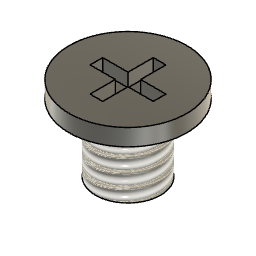
PSD Sun Sensor (Autodesk Fusion 360 archive; units mm, degrees)
design "M2x2 D3.5x0.5"
Autodesk Fusion 360 part; units mm, degrees
sketch "Sketch1" plane through (0, 0, 0) normal (0, 0, 1) x (1, 0, 0)
  circle A0 centre (0, 0) radius 1
  dimension "d1" = 2
  constraint coincident A0.centre origin
  measures "d1" diameter of A0
extrude "Extrude1" add sketch "Sketch1" against normal blind 2
sketch "Sketch2" plane through (0, 0, 0) normal (0, 0, 1) x (1, 0, 0)
  circle A0 centre (0, 0) radius 1.75
  dimension "d4" = 3.5
  constraint coincident A0.centre origin
  measures "d4" diameter of A0
extrude "Extrude2" add sketch "Sketch2" along normal blind 0.5
thread "Thread1" "ISO Metric profile 2.0 M2x0.4 6g" major diameter 1.9335 minor diameter 1.478 pitch 0.4 angle 60 resizes the face on face at (0.9988, -0.0498, -1.3333)
sketch "Sketch3" plane through (0, 0, 0.5) normal (0, 0, 1) x (-1, 0, 0)
  circle A0 centre (0, 0) radius 1.75
  line L0 (-0.9401, -0.188) -> (0.9401, -0.188)
  line L1 (0.9401, -0.188) -> (0.9401, 0.188)
  line L2 (0.9401, 0.188) -> (-0.9401, 0.188)
  line L3 (-0.9401, 0.188) -> (-0.9401, -0.188)
  line L4 (-0.9401, -0.188) -> (0.9401, 0.188) construction
  line L5 (0.9401, -0.188) -> (-0.9401, 0.188) construction
  line L6 (-0.188, -0.9401) -> (0.188, -0.9401)
  line L7 (0.188, -0.9401) -> (0.188, 0.9401)
  line L8 (0.188, 0.9401) -> (-0.188, 0.9401)
  line L9 (-0.188, 0.9401) -> (-0.188, -0.9401)
  line L10 (-0.188, -0.9401) -> (0.188, 0.9401) construction
  line L11 (0.188, -0.9401) -> (-0.188, 0.9401) construction
  constraint horizontal L0
  constraint perpendicular L0 L1
  constraint parallel L0 L2
  constraint parallel L1 L3
  constraint coincident L4 A0.centre
  constraint coincident L5 A0.centre
  constraint coincident A0.centre origin
  constraint horizontal L6
  constraint perpendicular L6 L7
  constraint parallel L6 L8
  constraint parallel L7 L9
  constraint coincident L10 A0.centre
  constraint coincident L11 A0.centre
  constraint equal L3 L6
  constraint equal L0 L9
extrude "Extrude3" cut sketch "Sketch3" against normal blind 0.4 contours L0 L2 L3 L9 | L0 L2 L7 L9 | L0 L6 L7 L9 | L0 L1 L2 L7 | L2 L7 L8 L9

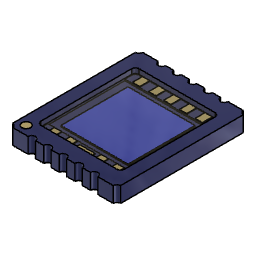
design "Hamamatsu S5990-01"
Autodesk Fusion 360 part; units mm, degrees
sketch "Sketch1" plane through (0, 0, 0) normal (0, 0, 1) x (1, 0, 0)
  line L0 (4.4, 5.3) -> (-4.4, 5.3)
  line L1 (-4.4, 5.3) -> (-4.4, -5.3)
  line L2 (-4.4, -5.3) -> (4.4, -5.3)
  line L3 (4.4, -5.3) -> (4.4, 5.3)
  line L4 (4.4, 5.3) -> (-4.4, -5.3) construction
  line L5 (-4.4, 5.3) -> (4.4, -5.3) construction
  circle A0 centre (-4.4, 5.3) radius 0.3
  circle A1 centre (4.4, 5.3) radius 0.3
  circle A2 centre (-4.4, -5.3) radius 0.3
  circle A3 centre (4.4, -5.3) radius 0.3
  dimension "d1" = 8.8
  dimension "d2" = 10.6
  dimension "d3" = 0.6
  constraint horizontal L0
  constraint perpendicular L0 L1
  constraint parallel L0 L2
  constraint parallel L1 L3
  constraint coincident L4 origin
  constraint coincident L5 origin
  constraint coincident L0.end L1.start
  constraint coincident L0.start L3.end
  constraint coincident L1.end L2.start
  constraint coincident L2.end L3.start
  constraint equal A1 A3
  constraint equal A2 A3
  constraint equal A0 A2
  measures "d1" distance of L1.end L2.end
  measures "d2" distance of L0.end L1.end
  measures "d3" diameter of A0
extrude "Extrude1" add sketch "Sketch1" along normal blind 1.26 contours L0 L1 L2 L3 A0 A1 A2 A3 makes body 1
sketch "Sketch2" plane through (0, 0, 1.26) normal (0, 0, 1) x (-1, 0, 0)
  line L0 (4.4, -5) -> (4.4, 5)
  arc A0 (4.1, 5.3) -> (4.4, 5) centre (4.4, 5.3) ccw
  line L1 (4.1, 5.3) -> (-4.1, 5.3)
  arc A1 (-4.4, 5) -> (-4.1, 5.3) centre (-4.4, 5.3) ccw
  line L2 (-4.4, 5) -> (-4.4, -5)
  arc A2 (-4.1, -5.3) -> (-4.4, -5) centre (-4.4, -5.3) ccw
  line L3 (-4.1, -5.3) -> (4.1, -5.3)
  arc A3 (4.4, -5) -> (4.1, -5.3) centre (4.4, -5.3) ccw
  line L4 (-3.4, -4) -> (3.4, -4)
  line L5 (3.4, -4) -> (3.4, 4)
  line L6 (3.4, 4) -> (-3.4, 4)
  line L7 (-3.4, 4) -> (-3.4, -4)
  line L8 (-3.4, -4) -> (3.4, 4) construction
  line L9 (3.4, -4) -> (-3.4, 4) construction
  dimension "d6" = 1
  dimension "d7" = 1.3
  constraint horizontal L4
  constraint perpendicular L4 L5
  constraint parallel L4 L6
  constraint parallel L5 L7
  constraint coincident L8 origin
  constraint coincident L9 origin
  measures "d6" distance of L0 L5
  measures "d7" distance of L3 L4
extrude "Extrude2" cut sketch "Sketch2" against normal blind 0.46 contours L4 L5 L6 L7 bodies 1
sketch "Sketch3" plane through (0, 0, 0.8) normal (0, 0, 1) x (-1, 0, 0)
  line L0 (-3.4, 4) -> (-3.4, -4)
  line L1 (-3.4, -4) -> (3.4, -4)
  line L2 (3.4, -4) -> (3.4, 4)
  line L3 (3.4, 4) -> (-3.4, 4)
  line L4 (-3.4, -3.1358) -> (3.4, -3.1358)
  line L5 (3.4, -3.1358) -> (3.4, 3.1358)
  line L6 (3.4, 3.1358) -> (-3.4, 3.1358)
  line L7 (-3.4, 3.1358) -> (-3.4, -3.1358)
  line L8 (-3.4, -3.1358) -> (3.4, 3.1358) construction
  line L9 (3.4, -3.1358) -> (-3.4, 3.1358) construction
  constraint horizontal L4
  constraint perpendicular L4 L5
  constraint parallel L4 L6
  constraint parallel L5 L7
  constraint coincident L8 origin
  constraint coincident L9 origin
  constraint coincident L0 L4.start
sketch "Sketch6" plane through (0, 0, 0.8) normal (0, 0, 1) x (-1, 0, 0)
  line L0 (-3.4, 4) -> (-3.4, -4)
  line L1 (-3.4, -4) -> (3.4, -4)
  line L2 (3.4, -4) -> (3.4, 4)
  line L3 (3.4, 4) -> (-3.4, 4)
  line L4 (2.8165, -4) -> (2.2221, -4)
  line L5 (2.2221, -4) -> (2.2221, -3.1841)
  line L6 (2.2221, -3.1841) -> (2.8165, -3.1841)
  line L7 (2.8165, -3.1841) -> (2.8165, -4)
  line L8 (1.5027, -4) -> (0.9082, -4)
  line L9 (0.9082, -4) -> (0.9082, -3.1841)
  line L10 (0.9082, -3.1841) -> (1.5027, -3.1841)
  line L11 (1.5027, -3.1841) -> (1.5027, -4)
  line L12 (0.2802, -4) -> (-0.3143, -4)
  line L13 (-0.3143, -4) -> (-0.3143, -3.1841)
  line L14 (-0.3143, -3.1841) -> (0.2802, -3.1841)
  line L15 (0.2802, -3.1841) -> (0.2802, -4)
  line L16 (-1.007, -4) -> (-1.6015, -4)
  line L17 (-1.6015, -4) -> (-1.6015, -3.1841)
  line L18 (-1.6015, -3.1841) -> (-1.007, -3.1841)
  line L19 (-1.007, -3.1841) -> (-1.007, -4)
  line L20 (-2.2803, -4) -> (-2.8747, -4)
  line L21 (-2.8747, -4) -> (-2.8747, -3.1841)
  line L22 (-2.8747, -3.1841) -> (-2.2803, -3.1841)
  line L23 (-2.2803, -3.1841) -> (-2.2803, -4)
  line L24 (2.8085, 4) -> (2.2141, 4)
  line L25 (2.2141, 4) -> (2.2141, 3.1841)
  line L26 (2.2141, 3.1841) -> (2.8085, 3.1841)
  line L27 (2.8085, 3.1841) -> (2.8085, 4)
  line L28 (1.5132, 4) -> (0.9187, 4)
  line L29 (0.9187, 4) -> (0.9187, 3.1841)
  line L30 (0.9187, 3.1841) -> (1.5132, 3.1841)
  line L31 (1.5132, 3.1841) -> (1.5132, 4)
  line L32 (-1.0056, 4) -> (-1.6, 4)
  line L33 (-1.6, 4) -> (-1.6, 3.1841)
  line L34 (-1.6, 3.1841) -> (-1.0056, 3.1841)
  line L35 (-1.0056, 3.1841) -> (-1.0056, 4)
  line L36 (0.5753, 4) -> (-0.7, 4)
  line L37 (-0.7, 4) -> (-0.7, 3.3622)
  line L38 (-0.7, 3.3622) -> (0.5753, 3.3622)
  line L39 (0.5753, 3.3622) -> (0.5753, 4)
  line L40 (-2.2961, 4) -> (-2.8905, 4)
  line L41 (-2.8905, 4) -> (-2.8905, 3.1841)
  line L42 (-2.8905, 3.1841) -> (-2.2961, 3.1841)
  line L43 (-2.2961, 3.1841) -> (-2.2961, 4)
  constraint horizontal L4
  constraint vertical L5
  constraint horizontal L6
  constraint vertical L7
  constraint coincident L1 L4.start
  constraint horizontal L8
  constraint vertical L9
  constraint horizontal L10
  constraint vertical L11
  constraint coincident L1 L8.start
  constraint horizontal L12
  constraint vertical L13
  constraint horizontal L14
  constraint vertical L15
  constraint coincident L1 L12.start
  constraint horizontal L16
  constraint vertical L17
  constraint horizontal L18
  constraint vertical L19
  constraint coincident L1 L16.start
  constraint horizontal L20
  constraint vertical L21
  constraint horizontal L22
  constraint vertical L23
  constraint coincident L1 L20.start
  constraint equal L19 L23
  constraint equal L15 L19
  constraint equal L11 L15
  constraint equal L7 L11
  constraint equal L6 L10
  constraint equal L10 L14
  constraint equal L14 L18
  constraint equal L18 L22
  constraint horizontal L24
  constraint vertical L25
  constraint horizontal L26
  constraint vertical L27
  constraint coincident L3 L24.start
  constraint horizontal L28
  constraint vertical L29
  constraint horizontal L30
  constraint vertical L31
  constraint coincident L3 L28.start
  constraint horizontal L32
  constraint vertical L33
  constraint horizontal L34
  constraint vertical L35
  constraint coincident L3 L32.start
  constraint horizontal L36
  constraint vertical L37
  constraint horizontal L38
  constraint vertical L39
  constraint coincident L3 L36.start
  constraint horizontal L40
  constraint vertical L41
  constraint horizontal L42
  constraint vertical L43
  constraint coincident L3 L40.start
  constraint equal L34 L42
  constraint equal L30 L42
  constraint equal L26 L30
  constraint equal L6 L26
  constraint equal L27 L31
  constraint equal L7 L31
  constraint equal L7 L35
  constraint equal L35 L43
extrude "Extrude1'" add sketch "Sketch6" along normal blind 0.05 separate body contours L3 L40 L41 L42 L43 | L1 L20 L21 L22 L23 | L3 L32 L33 L34 L35 | L1 L16 L17 L18 L19 | L3 L36 L37 L38 L39 | L1 L12 L13 L14 L15 | L3 L28 L29 L30 L31 | L1 L8 L9 L10 L11 | L3 L24 L25 L26 L27 | L1 L4 L5 L6 L7 makes body 2 at (-0.082, 3.728, 0.8) makes body 3 at (1.4019, -3.728, 0.8) makes body 4 at (-2.4123, -3.728, 0.8) makes body 5 at (2.4942, -3.728, 0.8) makes body 6 at (-1.1064, 3.4561, 0.8) makes body 7 at (1.4033, 3.4561, 0.8) makes body 8 at (0.2749, -3.7874, 0.8) makes body 9 at (-1.315, -3.4561, 0.8) makes body 10 at (2.6765, 3.4561, 0.8) makes body 11 at (-2.4202, 3.4561, 0.8) in component "Component"
extrude "Extrude3" cut sketch "Sketch3" against normal blind 0.1 contours L0 L2 L4 L5 L6 L7 bodies 1
sketch "Sketch4" plane through (0, 0, 0.7) normal (0, 0, 1) x (-1, 0, 0)
  line L0 (-3.4, 3.1358) -> (-3.4, -3.1358)
  line L1 (-3.4, -3.1358) -> (3.4, -3.1358)
  line L2 (3.4, -3.1358) -> (3.4, 3.1358)
  line L3 (3.4, 3.1358) -> (-3.4, 3.1358)
  line L4 (-2.734, -2.734) -> (2.734, -2.734)
  line L5 (2.734, -2.734) -> (2.734, 2.734)
  line L6 (2.734, 2.734) -> (-2.734, 2.734)
  line L7 (-2.734, 2.734) -> (-2.734, -2.734)
  line L8 (-2.734, -2.734) -> (2.734, 2.734) construction
  line L9 (2.734, -2.734) -> (-2.734, 2.734) construction
  constraint horizontal L4
  constraint perpendicular L4 L5
  constraint parallel L4 L6
  constraint parallel L5 L7
  constraint coincident L8 origin
  constraint coincident L9 origin
  constraint equal L4 L5
extrude "Extrude1''" add sketch "Sketch4" along normal blind 0.1 separate body contours L4 L5 L6 L7 makes body 12 in component "Diode"
fillet "Fillet1" radius 0.3 4 edges at (-3.4, 4, 1.03) (-3.4, -4, 1.03) (3.4, -4, 1.03) (3.4, 4, 1.03) on bodies 1
sketch "Sketch5" plane through (0, 0, 0) normal (0, 0, 1) x (1, 0, 0)
  line L0 (4.4, 5.3) -> (-4.4, 5.3)
  line L1 (-4.4, 5.3) -> (-4.4, -5.3)
  line L2 (-4.4, -5.3) -> (4.4, -5.3)
  line L3 (4.4, -5.3) -> (4.4, 5.3)
  circle A0 centre (0, 5.3) radius 0.3
  circle A1 centre (1.27, 5.3) radius 0.3
  circle A2 centre (2.54, 5.3) radius 0.3
  circle A3 centre (-1.27, 5.3) radius 0.3
  circle A4 centre (-2.54, 5.3) radius 0.3
  circle A5 centre (0, -5.3) radius 0.3
  circle A6 centre (1.27, -5.3) radius 0.3
  circle A7 centre (2.54, -5.3) radius 0.3
  circle A8 centre (-1.27, -5.3) radius 0.3
  circle A9 centre (-2.54, -5.3) radius 0.3
  line L4 (-2.84, 5.3) -> (-2.24, 5.3)
  line L5 (-2.24, 5.3) -> (-2.24, 3.8)
  line L6 (-2.24, 3.8) -> (-2.84, 3.8)
  line L7 (-2.84, 3.8) -> (-2.84, 5.3)
  line L8 (-1.57, 5.3) -> (-0.97, 5.3)
  line L9 (-0.97, 5.3) -> (-0.97, 3.8)
  line L10 (-0.97, 3.8) -> (-1.57, 3.8)
  line L11 (-1.57, 3.8) -> (-1.57, 5.3)
  line L12 (-0.3, 5.3) -> (0.3, 5.3)
  line L13 (0.3, 5.3) -> (0.3, 3.8)
  line L14 (0.3, 3.8) -> (-0.3, 3.8)
  line L15 (-0.3, 3.8) -> (-0.3, 5.3)
  line L16 (0.97, 5.3) -> (1.57, 5.3)
  line L17 (1.57, 5.3) -> (1.57, 3.8)
  line L18 (1.57, 3.8) -> (0.97, 3.8)
  line L19 (0.97, 3.8) -> (0.97, 5.3)
  line L20 (2.24, 5.3) -> (2.84, 5.3)
  line L21 (2.84, 5.3) -> (2.84, 3.8)
  line L22 (2.84, 3.8) -> (2.24, 3.8)
  line L23 (2.24, 3.8) -> (2.24, 5.3)
  line L24 (-2.84, -5.3) -> (-2.24, -5.3)
  line L25 (-2.24, -5.3) -> (-2.24, -3.8)
  line L26 (-2.24, -3.8) -> (-2.84, -3.8)
  line L27 (-2.84, -3.8) -> (-2.84, -5.3)
  line L28 (-1.57, -5.3) -> (-0.97, -5.3)
  line L29 (-0.97, -5.3) -> (-0.97, -3.8)
  line L30 (-0.97, -3.8) -> (-1.57, -3.8)
  line L31 (-1.57, -3.8) -> (-1.57, -5.3)
  line L32 (-0.3, -5.3) -> (0.3, -5.3)
  line L33 (0.3, -5.3) -> (0.3, -2.8)
  line L34 (0.3, -2.8) -> (-0.3, -2.8)
  line L35 (-0.3, -2.8) -> (-0.3, -5.3)
  line L36 (0.97, -5.3) -> (1.57, -5.3)
  line L37 (1.57, -5.3) -> (1.57, -3.8)
  line L38 (1.57, -3.8) -> (0.97, -3.8)
  line L39 (0.97, -3.8) -> (0.97, -5.3)
  line L40 (2.24, -5.3) -> (2.84, -5.3)
  line L41 (2.84, -5.3) -> (2.84, -3.8)
  line L42 (2.84, -3.8) -> (2.24, -3.8)
  line L43 (2.24, -3.8) -> (2.24, -5.3)
  dimension "d17" = 0.6
  dimension "d18" = 1.27
  dimension "d19" = 1.27
  dimension "d20" = 1.27
  dimension "d21" = 1.27
  dimension "d22" = 1.27
  dimension "d23" = 1.27
  dimension "d24" = 1.27
  dimension "d25" = 1.27
  dimension "d26" = 1.5
  dimension "d38" = 2.5
  constraint midpoint L0 A0.centre
  constraint coincident L0 A1.centre
  constraint coincident L0 A2.centre
  constraint coincident L0 A3.centre
  constraint coincident L0 A4.centre
  constraint midpoint L2 A5.centre
  constraint coincident L2 A6.centre
  constraint coincident L2 A7.centre
  constraint coincident L2 A8.centre
  constraint coincident L2 A9.centre
  constraint equal A8 A9
  constraint equal A5 A9
  constraint equal A5 A6
  constraint equal A6 A7
  constraint equal A2 A7
  constraint equal A1 A2
  constraint equal A1 A3
  constraint equal A3 A4
  constraint equal A0 A4
  constraint perpendicular L4 L5
  constraint parallel L4 L6
  constraint parallel L5 L7
  constraint coincident A4 L4.end
  constraint coincident L0 L4.end
  constraint parallel L0 L4
  constraint coincident A4 L4.start
  constraint perpendicular L8 L9
  constraint parallel L8 L10
  constraint parallel L9 L11
  constraint coincident A3 L8.end
  constraint coincident L0 L8.end
  constraint perpendicular L7 L8
  constraint coincident A3 L8.start
  constraint perpendicular L12 L13
  constraint parallel L12 L14
  constraint parallel L13 L15
  constraint coincident A0 L12.end
  constraint coincident L0 L12.end
  constraint perpendicular L9 L12
  constraint coincident A0 L12.start
  constraint perpendicular L16 L17
  constraint parallel L16 L18
  constraint parallel L17 L19
  constraint coincident L0 L16.end
  constraint coincident A1 L16.end
  constraint perpendicular L13 L16
  constraint coincident A1 L16.start
  constraint perpendicular L20 L21
  constraint parallel L20 L22
  constraint parallel L21 L23
  constraint coincident A2 L20.end
  constraint coincident L0 L20.end
  constraint perpendicular L17 L20
  constraint coincident A2 L20.start
  constraint perpendicular L24 L25
  constraint parallel L24 L26
  constraint parallel L25 L27
  constraint coincident A9 L24.end
  constraint coincident L2 L24.end
  constraint perpendicular L23 L24
  constraint coincident A9 L24.start
  constraint perpendicular L28 L29
  constraint parallel L28 L30
  constraint parallel L29 L31
  constraint coincident A8 L28.end
  constraint coincident L2 L28.end
  constraint perpendicular L27 L28
  constraint coincident A8 L28.start
  constraint perpendicular L32 L33
  constraint parallel L32 L34
  constraint parallel L33 L35
  constraint coincident A5 L32.end
  constraint coincident L2 L32.end
  constraint perpendicular L29 L32
  constraint coincident A5 L32.start
  constraint perpendicular L36 L37
  constraint parallel L36 L38
  constraint parallel L37 L39
  constraint coincident A6 L36.end
  constraint coincident L2 L36.end
  constraint perpendicular L33 L36
  constraint coincident A6 L36.start
  constraint perpendicular L40 L41
  constraint parallel L40 L42
  constraint parallel L41 L43
  constraint coincident A7 L40.end
  constraint coincident L2 L40.end
  constraint perpendicular L39 L40
  constraint coincident A7 L40.start
  constraint equal L7 L11
  constraint equal L11 L19
  constraint equal L19 L23
  constraint equal L23 L27
  constraint equal L27 L31
  constraint equal L39 L43
  constraint equal L11 L15
  constraint equal L31 L39
  measures "d17" diameter of A0
  measures "d18" distance of A0.centre A3.centre
  measures "d19" distance of A0.centre A1.centre
  measures "d20" distance of A1.centre A2.centre
  measures "d21" distance of A3.centre A4.centre
  measures "d22" distance of A5.centre A8.centre
  measures "d23" distance of A8.centre A9.centre
  measures "d24" distance of A5.centre A6.centre
  measures "d25" distance of A6.centre A7.centre
  measures "d26" distance of A4.centre L6
  measures "d38" distance of A5.centre L34
extrude "Extrude5" cut sketch "Sketch5" along normal blind 1.5 contours L0 A2 L20 | L2 A7 L40 | L0 A1 L16 | L2 A6 L36 | L0 A0 L12 | L2 A5 L32 | L0 A3 L8 | L2 A8 L28 | L0 A4 L4 | L2 A9 L24 picked at (2.5697, 5.1028) picked at (2.6301, -5.2566) picked at (1.2077, 5.2218) picked at (1.3433, -5.232) picked at (-0.0623, 5.2218) picked at (-0.0989, -5.2851) picked at (-1.3323, 5.2218) picked at (-1.1967, -5.232) picked at (-2.5103, 5.1028) picked at (-2.4499, -5.2566) bodies 1
extrude "Extrude1'''" add sketch "Sketch2" against normal blind 0.4 separate body contours L4 L5 L6 L7 makes body 13 in component "Resin Window"
fillet "Fillet1'" radius 0.3 4 edges at (-3.4, -4, 1.06) (3.4, -4, 1.06) (3.4, 4, 1.06) (-3.4, 4, 1.06) on bodies 13 in component "Resin Window"
sketch "Sketch7" plane through (0, 0, 1.26) normal (0, 0, 1) x (-1, 0, 0)
  arc A0 (0.3, -5.3) -> (-0.3, -5.3) centre (0, -5.3) ccw
  line L0 (0.3, -5.3) -> (0.97, -5.3)
  arc A1 (1.57, -5.3) -> (0.97, -5.3) centre (1.27, -5.3) ccw
  line L1 (1.57, -5.3) -> (2.24, -5.3)
  arc A2 (2.84, -5.3) -> (2.24, -5.3) centre (2.54, -5.3) ccw
  line L2 (2.84, -5.3) -> (4.1, -5.3)
  arc A3 (4.4, -5) -> (4.1, -5.3) centre (4.4, -5.3) ccw
  line L3 (4.4, -5) -> (4.4, 5)
  arc A4 (4.1, 5.3) -> (4.4, 5) centre (4.4, 5.3) ccw
  line L4 (4.1, 5.3) -> (2.84, 5.3)
  arc A5 (2.24, 5.3) -> (2.84, 5.3) centre (2.54, 5.3) ccw
  line L5 (2.24, 5.3) -> (1.57, 5.3)
  arc A6 (0.97, 5.3) -> (1.57, 5.3) centre (1.27, 5.3) ccw
  line L6 (0.97, 5.3) -> (0.3, 5.3)
  arc A7 (-0.3, 5.3) -> (0.3, 5.3) centre (0, 5.3) ccw
  line L7 (-0.3, 5.3) -> (-0.97, 5.3)
  arc A8 (-1.57, 5.3) -> (-0.97, 5.3) centre (-1.27, 5.3) ccw
  line L8 (-1.57, 5.3) -> (-2.24, 5.3)
  arc A9 (-2.84, 5.3) -> (-2.24, 5.3) centre (-2.54, 5.3) ccw
  line L9 (-2.84, 5.3) -> (-4.1, 5.3)
  arc A10 (-4.4, 5) -> (-4.1, 5.3) centre (-4.4, 5.3) ccw
  line L10 (-4.4, 5) -> (-4.4, -5)
  arc A11 (-4.1, -5.3) -> (-4.4, -5) centre (-4.4, -5.3) ccw
  line L11 (-4.1, -5.3) -> (-2.84, -5.3)
  arc A12 (-2.24, -5.3) -> (-2.84, -5.3) centre (-2.54, -5.3) ccw
  line L12 (-2.24, -5.3) -> (-1.57, -5.3)
  arc A13 (-0.97, -5.3) -> (-1.57, -5.3) centre (-1.27, -5.3) ccw
  line L13 (-0.97, -5.3) -> (-0.3, -5.3)
  line L14 (-0.3, -5.3) -> (-0.3, -5.3)
  line L15 (3.1, -4) -> (-3.1, -4)
  arc A14 (-3.4, -3.7) -> (-3.1, -4) centre (-3.1, -3.7) ccw
  line L16 (-3.4, -3.7) -> (-3.4, 3.7)
  arc A15 (-3.1, 4) -> (-3.4, 3.7) centre (-3.1, 3.7) ccw
  line L17 (-3.1, 4) -> (3.1, 4)
  arc A16 (3.4, 3.7) -> (3.1, 4) centre (3.1, 3.7) ccw
  line L18 (3.4, 3.7) -> (3.4, -3.7)
  arc A17 (3.1, -4) -> (3.4, -3.7) centre (3.1, -3.7) ccw
  circle A18 centre (3.7, 4.6) radius 0.35
  line L19 (4.4, 5.3) -> (-4.4, 5.3)
  line L20 (4.4, -5.3) -> (4.4, 5.3)
  dimension "d39" = 0.7
  dimension "d40" = 0.7
  dimension "d41" = 0.7
  measures "d39" distance of A18.centre L20
  measures "d40" distance of A18.centre L19
  measures "d41" diameter of A18
extrude "Extrude1''''" add sketch "Sketch7" along normal blind 0.02 separate body contours A18 makes body 14 in component "Index Mark"
extrude "Extrude1'''''" add sketch "Sketch5" against normal blind 0.02 separate body contours A2 L21 L22 L23 | A7 L41 L42 L43 | A1 L17 L18 L19 | A6 L37 L38 L39 | A0 L13 L14 L15 | A5 L33 L34 L35 | A3 L9 L10 L11 | A8 L29 L30 L31 | A4 L5 L6 L7 | A9 L25 L26 L27 makes body 15 at (-0.0075, 4.2003, 0) makes body 16 at (1.2625, -4.2003, 0) makes body 17 at (-2.5475, -4.2003, 0) makes body 18 at (2.5325, -4.2003, 0) makes body 19 at (1.2775, 4.2003, 0) makes body 20 at (-1.2625, 4.2003, 0) makes body 21 at (-0.0075, -3.5336, 0) makes body 22 at (-1.2775, -4.2003, 0) makes body 23 at (-2.5325, 4.2003, 0) makes body 24 at (2.5475, 4.2003, 0) in component "Component'"
component "Component" placed x (1, 0, 0) y (0, 1, 0) z (0, 0, 1) at (0, 0, 0)
component "Diode" placed x (1, 0, 0) y (0, 1, 0) z (0, 0, 1) at (0, 0, 0)
component "Resin Window" placed x (1, 0, 0) y (0, 1, 0) z (0, 0, 1) at (0, 0, 0)
component "Index Mark" placed x (1, 0, 0) y (0, 1, 0) z (0, 0, 1) at (0, 0, 0)
component "Component'" placed x (1, 0, 0) y (0, 1, 0) z (0, 0, 1) at (0, 0, 0)

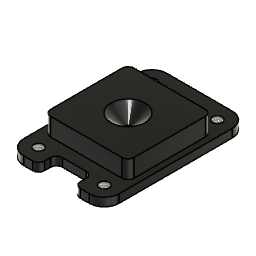
design "Cover"
Autodesk Fusion 360 part; units mm, degrees
sketch "Pinhole Geometry" plane through (0, 0, 0) normal (1, 0, 0) x (0, 1, 0)
  line L0 (-2, 0) -> (2, 0)
  line L1 (2, 0) -> (2, 0.8)
  line L2 (-2, 0.8) -> (-2, 0)
  line L3 (-2, 0.8) -> (-1.4384, 0.8)
  line L4 (-1.4384, 0.8) -> (1.4384, 0.8)
  line L5 (1.4384, 0.8) -> (2, 0.8)
  line L6 (0, 0) -> (0, 2.1426) construction
  line L7 (-0.4, 2.1426) -> (0.4, 2.1426)
  line L8 (-2, 0.8) -> (-0.4, 2.1426) construction
  line L9 (-0.4, 2.1426) -> (-0.4, 2.3426)
  line L10 (0.4, 2.1426) -> (0.4, 2.3426)
  line L11 (0.4, 2.3426) -> (-1.4384, 0.8) construction
  line L12 (-0.4, 2.3426) -> (0.4, 2.3426)
  line L13 (0.4, 2.3426) -> (2.852, 4.4)
  line L14 (-0.4, 2.3426) -> (-2.852, 4.4)
  line L15 (-2.852, 4.4) -> (2.852, 4.4)
  line L16 (0, 2.3426) -> (0, 4.4)
  line L17 (-0.4, 2.1426) -> (2.5317, 4.6025) construction
  line L18 (-1.7192, 0.8) -> (-1.7192, 0.7)
  line L19 (1.7192, 0.8) -> (1.7192, 0.7)
  line L20 (-0.4, 2.3426) -> (1.4384, 0.8) construction
  line L21 (0.4, 2.1426) -> (2, 0.8) construction
  line L22 (0, 2.2426) -> (0, 2.3426)
  line L23 (0, 2.2426) -> (0, 2.1426)
  line L24 (-0.4, 2.1426) -> (-4, 2.1426)
  line L25 (-2.852, 4.4) -> (-4, 4.4)
  line L26 (-4, 4.4) -> (-4, 2.1426)
  line L27 (0.4, 2.1426) -> (4, 2.1426)
  line L28 (4, 2.1426) -> (4, 4.4)
  line L29 (4, 4.4) -> (2.852, 4.4)
  line L30 (0.4, 2.1426) -> (-2.5007, 4.5765) construction
  dimension "d41" = 4
  dimension "d44" = 0.8
  dimension "d48" = 0.2
  dimension "d49" = 4.4
  dimension "d52" = 0.8
  dimension "d53" = 50
  dimension "d55" = 0.5616
  dimension "d56" = 2.1426
  dimension "d57" = 2.2574
  dimension "d58" = 3.4384
  dimension "d60" = 1.4426
  constraint horizontal L0
  constraint vertical L1
  constraint vertical L2
  constraint midpoint L6.start L0
  constraint perpendicular L2 L3
  constraint parallel L3 L4
  constraint perpendicular L1 L5
  constraint coincident L6.start origin
  constraint vertical L6
  constraint midpoint L6.end L7
  constraint equal L3 L5
  constraint perpendicular L7 L9
  constraint perpendicular L7 L10
  constraint horizontal L15
  constraint equal L13 L14
  constraint horizontal L12
  constraint parallel L11 L13
  constraint midpoint L12 L16.start
  constraint midpoint L15 L16.end
  constraint parallel L13 L17
  constraint parallel L8 L11
  constraint midpoint L3 L18.start
  constraint perpendicular L3 L18
  constraint midpoint L5 L19.start
  constraint perpendicular L5 L19
  constraint perpendicular L12 L22
  constraint perpendicular L7 L23
  constraint equal L22 L23
  constraint perpendicular L9 L24
  constraint parallel L15 L25
  constraint perpendicular L24 L26
  constraint perpendicular L10 L27
  constraint perpendicular L7 L28
  constraint equal L24 L27
  constraint horizontal L29
  constraint parallel L21 L30
  measures "d41" distance of L1 L2
  measures "d44" distance of L7.start L7.end
  measures "d48" distance of L7 L12
  measures "d49" distance of L6.start L15
  measures "d52" distance of L0.start L2.start
  measures "d53" angle of L13 L16
  measures "d55" distance of L2.start L3.end
  measures "d56" distance of L6.start L7
  measures "d57" distance of L7 L15
  measures "d58" distance of L18.start L19.start
  measures "d60" distance of L4 L22.start
sketch "Outline" plane through (0, 0, 0) normal (0, 0, 1) x (1, 0, 0)
  line L0 (8, 12) -> (-8, 12)
  line L1 (-8, 12) -> (-8, -12)
  line L2 (-8, -12) -> (8, -12)
  line L3 (8, -12) -> (8, 12)
  line L4 (8, 12) -> (-8, -12) construction
  line L5 (-8, 12) -> (8, -12) construction
  dimension "d1" = 16
  dimension "d2" = 24
  constraint horizontal L0
  constraint perpendicular L0 L1
  constraint parallel L0 L2
  constraint parallel L1 L3
  constraint coincident L4 origin
  constraint coincident L5 origin
  measures "d1" distance of L1.end L2.end
  measures "d2" distance of L0.end L1.end
extrude "Extrude1" add sketch "Outline" along normal blind 1.4
sketch "Top" plane through (0, 0, 1.4) normal (0, 0, 1) x (-1, 0, 0)
  line L0 (-8, 12) -> (-8, -12)
  line L1 (-8, -12) -> (8, -12)
  line L2 (8, -12) -> (8, 12)
  line L3 (8, 12) -> (-8, 12)
  line L4 (-7, -7) -> (7, -7)
  line L5 (7, -7) -> (7, 7)
  line L6 (7, 7) -> (-7, 7)
  line L7 (-7, 7) -> (-7, -7)
  line L8 (-7, -7) -> (7, 7) construction
  line L9 (7, -7) -> (-7, 7) construction
  dimension "d5" = 14
  dimension "d6" = 14
  constraint horizontal L4
  constraint perpendicular L4 L5
  constraint parallel L4 L6
  constraint parallel L5 L7
  constraint coincident L8 origin
  constraint coincident L9 origin
  measures "d5" distance of L5.end L6.end
  measures "d6" distance of L4.end L5.end
extrude "Extrude2" add sketch "Top" along normal up to surface (3 mm away) contours L4 L5 L6 L7
sketch "Connector cut out" plane through (0, 0, 1.4) normal (0, 0, 1) x (-1, 0, 0)
  line L0 (-8, 12) -> (-8, -12)
  line L1 (-8, -12) -> (8, -12)
  line L2 (8, -12) -> (8, 12)
  line L3 (8, 12) -> (-8, 12)
  line L4 (8, 12) -> (-8, 12)
  line L5 (3, 12) -> (3, 9)
  line L6 (3, 9) -> (-3, 9)
  line L7 (3, 12) -> (-3, 12)
  line L8 (-3, 9) -> (-3, 12)
  line L9 (7, -7) -> (-7, -7)
  line L10 (-7, -7) -> (-7, 7)
  line L11 (-7, 7) -> (7, 7)
  line L12 (7, 7) -> (7, -7)
  dimension "d9" = 6
  dimension "d10" = 3
  constraint coincident L4 L5.start
  constraint perpendicular L4 L5
  constraint perpendicular L5 L6
  constraint coincident L4 L7.end
  constraint midpoint L3 L7
  constraint perpendicular L7 L8
  measures "d9" distance of L5 L8
  measures "d10" distance of L6 L7
extrude "Extrude3" cut sketch "Connector cut out" against normal through all contours L3 L4 L5 L6 L7 L8
fillet "Fillet1" radius 2.5 4 edges at (-8, 12, 0.7) (8, 12, 0.7) (8, -12, 0.7) (-8, -12, 0.7)
fillet "Fillet1" radius 1 4 edges at (-3, -9, 0.7) (-3, -12, 0.7) (3, -9, 0.7) (3, -12, 0.7)
fillet "Fillet1" radius 1 4 edges at (-7, -7, 2.9) (-7, 7, 2.9) (7, 7, 2.9) (7, -7, 2.9)
sketch "Attachment holes" plane through (0, 0, 0) normal (0, 0, -1) x (1, 0, 0)
  arc A0 (4, 12) -> (3, 11) centre (4, 11) ccw
  line L0 (3, 11) -> (3, 10)
  arc A1 (2, 9) -> (3, 10) centre (2, 10) ccw
  line L1 (2, 9) -> (-2, 9)
  arc A2 (-3, 10) -> (-2, 9) centre (-2, 10) ccw
  line L2 (-3, 10) -> (-3, 11)
  arc A3 (-3, 11) -> (-4, 12) centre (-4, 11) ccw
  line L3 (-4, 12) -> (-5.5, 12)
  arc A4 (-5.5, 12) -> (-8, 9.5) centre (-5.5, 9.5) ccw
  line L4 (-8, 9.5) -> (-8, -9.5)
  arc A5 (-8, -9.5) -> (-5.5, -12) centre (-5.5, -9.5) ccw
  line L5 (-5.5, -12) -> (5.5, -12)
  arc A6 (5.5, -12) -> (8, -9.5) centre (5.5, -9.5) ccw
  line L6 (8, -9.5) -> (8, 9.5)
  arc A7 (8, 9.5) -> (5.5, 12) centre (5.5, 9.5) ccw
  line L7 (5.5, 12) -> (4, 12)
  line L8 (5.5, 9.5) -> (-5.5, 9.5)
  line L9 (-5.5, 9.5) -> (-5.5, -9.5)
  line L10 (-5.5, -9.5) -> (5.5, -9.5)
  line L11 (5.5, -9.5) -> (5.5, 9.5)
  line L12 (5.5, 9.5) -> (-5.5, -9.5) construction
  line L13 (-5.5, 9.5) -> (5.5, -9.5) construction
  dimension "d18" = 11
  dimension "d19" = 19
  constraint horizontal L8
  constraint perpendicular L8 L9
  constraint parallel L8 L10
  constraint parallel L9 L11
  constraint coincident L12 origin
  constraint coincident L13 origin
  measures "d18" distance of A5.centre A6.centre
  measures "d19" distance of A4.centre A5.centre
hole "Hole1" at (5.5, -9.5, 0) at (-5.5, -9.5, 0) at (-5.5, 9.5, 0) at (5.5, 9.5, 0) direction (0, 0, 1) diameter 2 end through all
thread "Thread1" "ISO Metric profile 2.0 M2x0.4 6H" major diameter 2.074 minor diameter 1.623 pitch 0.4 angle 60 resizes the face on face at (5.5498, -8.5012, 0.4667) on face at (5.5498, 10.4988, 0.4667) on face at (-5.4502, -8.5012, 0.4667) on face at (-5.4502, 10.4988, 0.4667)
sketch "Sensor Cutout" plane through (0, 0, 0) normal (0, 0, -1) x (1, 0, 0)
  circle A0 centre (-5.5, -9.5) radius 0.8115
  circle A1 centre (5.5, 9.5) radius 0.8115
  circle A2 centre (-5.5, 9.5) radius 0.8115
  circle A3 centre (5.5, -9.5) radius 0.8115
  arc A4 (4, 12) -> (3, 11) centre (4, 11) ccw
  line L0 (3, 11) -> (3, 10)
  arc A5 (2, 9) -> (3, 10) centre (2, 10) ccw
  line L1 (2, 9) -> (-2, 9)
  arc A6 (-3, 10) -> (-2, 9) centre (-2, 10) ccw
  line L2 (-3, 10) -> (-3, 11)
  arc A7 (-3, 11) -> (-4, 12) centre (-4, 11) ccw
  line L3 (-4, 12) -> (-5.5, 12)
  arc A8 (-5.5, 12) -> (-8, 9.5) centre (-5.5, 9.5) ccw
  line L4 (-8, 9.5) -> (-8, -9.5)
  arc A9 (-8, -9.5) -> (-5.5, -12) centre (-5.5, -9.5) ccw
  line L5 (-5.5, -12) -> (5.5, -12)
  arc A10 (5.5, -12) -> (8, -9.5) centre (5.5, -9.5) ccw
  line L6 (8, -9.5) -> (8, 9.5)
  arc A11 (8, 9.5) -> (5.5, 12) centre (5.5, 9.5) ccw
  line L7 (5.5, 12) -> (4, 12)
  line L8 (5, 6) -> (-5, 6)
  line L9 (-5, 6) -> (-5, -6)
  line L10 (-5, -6) -> (5, -6)
  line L11 (5, -6) -> (5, 6)
  line L12 (5, 6) -> (-5, -6) construction
  line L13 (-5, 6) -> (5, -6) construction
  line L14 (-4.4, 5.3) -> (4.4, 5.3) construction
  line L15 (4.4, 5.3) -> (4.4, -5.3) construction
  line L16 (4.4, -5.3) -> (-4.4, -5.3) construction
  line L17 (-4.4, -5.3) -> (-4.4, 5.3) construction
  line L18 (-4.4, 5.3) -> (4.4, -5.3) construction
  line L19 (4.4, 5.3) -> (-4.4, -5.3) construction
  dimension "d23" = 10
  dimension "d24" = 12
  dimension "d39" = 8.8
  dimension "d40" = 10.6
  constraint horizontal L8
  constraint perpendicular L8 L9
  constraint parallel L8 L10
  constraint parallel L9 L11
  constraint coincident L12 origin
  constraint coincident L13 origin
  constraint horizontal L14
  constraint perpendicular L14 L15
  constraint parallel L14 L16
  constraint parallel L15 L17
  constraint coincident L18 origin
  constraint coincident L19 origin
  measures "d23" distance of L9.end L10.end
  measures "d24" distance of L8.end L9.end
  measures "d39" distance of L15.end L16.end
  measures "d40" distance of L14.end L15.end
extrude "Extrude4" cut sketch "Sensor Cutout" against normal up to surface (2.1426 mm away) contours L8 L9 L10 L11
fillet "Fillet2" radius 1 4 edges at (5, -6, 1.0713) (-5, -6, 1.0713) (-5, 6, 1.0713) (5, 6, 1.0713)
revolve "Revolve1" cut sketch "Pinhole Geometry" angle 360 about axis through (0, 0, 1.75) along (0, 0, 1) contours L7 L10 L12 L22 L23 | L12 L13 L15 L16
equation "hole_diameter = 0.8 mm"
equation "d44 = hole_diameter"

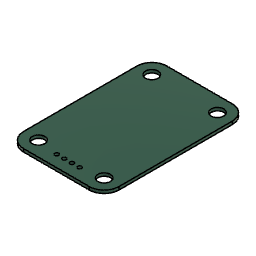
design "Simplfied PCB"
Autodesk Fusion 360 part; units mm, degrees
sketch "Outline" plane through (0, 0, 0) normal (0, 0, 1) x (1, 0, 0)
  line L0 (8, 12) -> (-8, 12)
  line L1 (-8, 12) -> (-8, -12)
  line L2 (-8, -12) -> (8, -12)
  line L3 (8, -12) -> (8, 12)
  line L4 (8, 12) -> (-8, -12) construction
  line L5 (-8, 12) -> (8, -12) construction
  dimension "d1" = 16
  dimension "d2" = 24
  constraint horizontal L0
  constraint perpendicular L0 L1
  constraint parallel L0 L2
  constraint parallel L1 L3
  constraint coincident L4 origin
  constraint coincident L5 origin
  measures "d1" distance of L1.end L2.end
  measures "d2" distance of L0.end L1.end
extrude "Extrude1" add sketch "Outline" along normal blind 0.5
fillet "Fillet1" radius 2.5 4 edges at (-8, 12, 0.25) (8, 12, 0.25) (8, -12, 0.25) (-8, -12, 0.25)
sketch "Holes" plane through (0, 0, 0.5) normal (0, 0, 1) x (-1, 0, 0)
  arc A0 (8, 9.5) -> (5.5, 12) centre (5.5, 9.5) ccw
  line L0 (5.5, 12) -> (-5.5, 12)
  arc A1 (-5.5, 12) -> (-8, 9.5) centre (-5.5, 9.5) ccw
  line L1 (-8, 9.5) -> (-8, -9.5)
  arc A2 (-8, -9.5) -> (-5.5, -12) centre (-5.5, -9.5) ccw
  line L2 (-5.5, -12) -> (5.5, -12)
  arc A3 (5.5, -12) -> (8, -9.5) centre (5.5, -9.5) ccw
  line L3 (8, -9.5) -> (8, 9.5)
  line L4 (-5.5, -9.5) -> (5.5, -9.5)
  line L5 (5.5, -9.5) -> (5.5, 9.5)
  line L6 (5.5, 9.5) -> (-5.5, 9.5)
  line L7 (-5.5, 9.5) -> (-5.5, -9.5)
  line L8 (-5.5, -9.5) -> (5.5, 9.5) construction
  line L9 (5.5, -9.5) -> (-5.5, 9.5) construction
  dimension "d7" = 11
  dimension "d8" = 19
  constraint horizontal L4
  constraint perpendicular L4 L5
  constraint parallel L4 L6
  constraint parallel L5 L7
  constraint coincident L8 origin
  constraint coincident L9 origin
  measures "d7" distance of A0.centre A1.centre
  measures "d8" distance of A3.centre A0.centre
hole "Hole1" at (-5.5, 9.5, 0.5) at (-5.5, -9.5, 0.5) at (5.5, -9.5, 0.5) at (5.5, 9.5, 0.5) direction (0, 0, -1) diameter 2.1 depth 0.966 tip angle 118
sketch "Sketch3" plane through (0, 0, 0.5) normal (0, 0, 1) x (-1, 0, 0)
  circle A0 centre (-5.5, 9.5) radius 1.05
  circle A1 centre (5.5, -9.5) radius 1.05
  circle A2 centre (5.5, 9.5) radius 1.05
  circle A3 centre (-5.5, -9.5) radius 1.05
  arc A4 (8, 9.5) -> (5.5, 12) centre (5.5, 9.5) ccw
  line L0 (5.5, 12) -> (-5.5, 12)
  arc A5 (-5.5, 12) -> (-8, 9.5) centre (-5.5, 9.5) ccw
  line L1 (-8, 9.5) -> (-8, -9.5)
  arc A6 (-8, -9.5) -> (-5.5, -12) centre (-5.5, -9.5) ccw
  line L2 (-5.5, -12) -> (5.5, -12)
  arc A7 (5.5, -12) -> (8, -9.5) centre (5.5, -9.5) ccw
  line L3 (8, -9.5) -> (8, 9.5)
  line L4 (1.905, 10.03) -> (0.635, 10.03)
  line L5 (0.635, 10.03) -> (-0.635, 10.03)
  line L6 (-0.635, 10.03) -> (-1.905, 10.03)
  line L7 (0, 12) -> (0, 10.03) construction
  dimension "d12" = 1.27
  dimension "d16" = 1.97
  constraint horizontal L4
  constraint parallel L4 L5
  constraint parallel L5 L6
  constraint midpoint L0 L7.start
  constraint midpoint L5 L7.end
  constraint equal L4 L5
  constraint equal L5 L6
  constraint perpendicular L5 L7
  measures "d12" distance of L4.start L4.end
  measures "d16" distance of L7.start L7.end
hole "Hole2" at (1.905, -10.03, 0.5) at (0.635, -10.03, 0.5) at (-0.635, -10.03, 0.5) at (-1.905, -10.03, 0.5) direction (0, 0, -1) diameter 0.65 end through all
